Autodesk Inventor part; units mm, degrees
(part 2 of 2)
  point P149 (-121, -15)
  point P150 (-116, -14)
  point P151 (-117, -15)
  point P152 (-112, -14)
  point P153 (-113, -15)
  point P154 (-108, -14)
  point P155 (-109, -15)
  point P156 (-104, -14)
  point P157 (-105, -15)
  point P158 (-100, -14)
  point P159 (-101, -15)
  point P160 (-96, -14)
  point P161 (-97, -15)
  point P162 (-92, -14)
  point P163 (-93, -15)
  point P164 (-88, -14)
  point P165 (-89, -15)
  point P166 (-84, -14)
  point P167 (-85, -15)
  point P168 (-80, -14)
  point P169 (-81, -15)
  point P170 (-76, -14)
  point P171 (-77, -15)
  point P172 (-72, -14)
  point P173 (-73, -15)
  point P174 (-68, -14)
  point P175 (-69, -15)
  point P176 (-64, -14)
  point P177 (-65, -15)
  point P178 (-60, -14)
  point P179 (-61, -15)
  point P180 (-56, -14)
  point P181 (-57, -15)
  point P182 (-52, -14)
  point P183 (-53, -15)
  point P184 (-48, -14)
  point P185 (-49, -15)
  point P186 (-44, -14)
  point P187 (-45, -15)
  point P188 (-40, -14)
  point P189 (-41, -15)
  point P190 (-36, -14)
  point P191 (-37, -15)
  point P192 (-32, -14)
  point P193 (-33, -15)
  point P194 (-124, -17)
  point P195 (-125, -18)
  point P196 (-120, -17)
  point P197 (-121, -18)
  point P198 (-116, -17)
  point P199 (-117, -18)
  dimension "d81" = 3
  dimension "d82" = 3
  dimension "d83" = 2
  dimension "d84" = 2
  dimension "d87" = 4
  dimension "d90" = 3
  constraints: 2304 end point, 2 collinear, 2 horizontal, 2 midpoint, 2 parallel, 1 perpendicular, 1 point on circle, 1 vertical, 2868 other
  measures "d81" distance from line of L4 point (-124, -5)
  measures "d82" horizontal distance of point (-128, -22.5) point (-125, -6)
  measures "d83" distance of L1.end L2.end
  measures "d84" distance of L0.end L1.end
  measures "d87" distance of L0.start L5.start
  measures "d90" distance of L0.start L97.start
extrude "Extrusion8" cut sketch "Sketch12" against normal blind 10
sketch "Sketch13" plane through (0, 2, 0) normal (0, 1, 0) x (1, 0, 0)
  point P0 (0, 0)
sketch "Sketch15" plane through (0, 2, 0) normal (0, 1, 0) x (1, 0, 0)
  line L0 (-29, -5) -> (-27, -5)
  line L1 (-27, -5) -> (-27, -7)
  line L2 (-27, -7) -> (-29, -7)
  line L3 (-29, -7) -> (-29, -5)
  line L4 (-31, -5) -> (-31, -7) projected
  line L5 (-25, -5) -> (-23, -5)
  line L6 (-23, -5) -> (-23, -7)
  line L7 (-23, -7) -> (-25, -7)
  line L8 (-25, -7) -> (-25, -5)
  line L9 (-21, -5) -> (-19, -5)
  line L10 (-19, -5) -> (-19, -7)
  line L11 (-19, -7) -> (-21, -7)
  line L12 (-21, -7) -> (-21, -5)
  line L13 (-29, -8) -> (-27, -8)
  line L14 (-27, -8) -> (-27, -10)
  line L15 (-27, -10) -> (-29, -10)
  line L16 (-29, -10) -> (-29, -8)
  line L17 (-25, -8) -> (-23, -8)
  line L18 (-23, -8) -> (-23, -10)
  line L19 (-23, -10) -> (-25, -10)
  line L20 (-25, -10) -> (-25, -8)
  line L21 (-21, -8) -> (-19, -8)
  line L22 (-19, -8) -> (-19, -10)
  line L23 (-19, -10) -> (-21, -10)
  line L24 (-21, -10) -> (-21, -8)
  line L25 (-29, -11) -> (-27, -11)
  line L26 (-27, -11) -> (-27, -13)
  line L27 (-27, -13) -> (-29, -13)
  line L28 (-29, -13) -> (-29, -11)
  line L29 (-25, -11) -> (-23, -11)
  line L30 (-23, -11) -> (-23, -13)
  line L31 (-23, -13) -> (-25, -13)
  line L32 (-25, -13) -> (-25, -11)
  line L33 (-21, -11) -> (-19, -11)
  line L34 (-19, -11) -> (-19, -13)
  line L35 (-19, -13) -> (-21, -13)
  line L36 (-21, -13) -> (-21, -11)
  line L37 (-29, -14) -> (-27, -14)
  line L38 (-27, -14) -> (-27, -16)
  line L39 (-27, -16) -> (-29, -16)
  line L40 (-29, -16) -> (-29, -14)
  line L41 (-25, -14) -> (-23, -14)
  line L42 (-23, -14) -> (-23, -16)
  line L43 (-23, -16) -> (-25, -16)
  line L44 (-25, -16) -> (-25, -14)
  line L45 (-21, -14) -> (-19, -14)
  line L46 (-19, -14) -> (-19, -16)
  line L47 (-19, -16) -> (-21, -16)
  line L48 (-21, -16) -> (-21, -14)
  line L49 (-29, -17) -> (-27, -17)
  line L50 (-27, -17) -> (-27, -19)
  line L51 (-27, -19) -> (-29, -19)
  line L52 (-29, -19) -> (-29, -17)
  line L53 (-25, -17) -> (-23, -17)
  line L54 (-23, -17) -> (-23, -19)
  line L55 (-23, -19) -> (-25, -19)
  line L56 (-25, -19) -> (-25, -17)
  line L57 (-21, -17) -> (-19, -17)
  line L58 (-19, -17) -> (-19, -19)
  line L59 (-19, -19) -> (-21, -19)
  line L60 (-21, -19) -> (-21, -17)
  line L61 (-29, -20) -> (-27, -20)
  line L62 (-27, -20) -> (-27, -22)
  line L63 (-27, -22) -> (-29, -22)
  line L64 (-29, -22) -> (-29, -20)
  line L65 (-25, -20) -> (-23, -20)
  line L66 (-23, -20) -> (-23, -22)
  line L67 (-23, -22) -> (-25, -22)
  line L68 (-25, -22) -> (-25, -20)
  line L69 (-21, -20) -> (-19, -20)
  line L70 (-19, -20) -> (-19, -22)
  line L71 (-19, -22) -> (-21, -22)
  line L72 (-21, -22) -> (-21, -20)
  line L73 (-29, -23) -> (-27, -23)
  line L74 (-27, -23) -> (-27, -25)
  line L75 (-27, -25) -> (-29, -25)
  line L76 (-29, -25) -> (-29, -23)
  line L77 (-25, -23) -> (-23, -23)
  line L78 (-23, -23) -> (-23, -25)
  line L79 (-23, -25) -> (-25, -25)
  line L80 (-25, -25) -> (-25, -23)
  line L81 (-21, -23) -> (-19, -23)
  line L82 (-19, -23) -> (-19, -25)
  line L83 (-19, -25) -> (-21, -25)
  line L84 (-21, -25) -> (-21, -23)
  line L85 (-29, -29) -> (-27, -29)
  line L86 (-27, -27) -> (-29, -27)
  line L87 (-29, -26) -> (-27, -26)
  line L88 (-27, -26) -> (-27, -28)
  line L89 (-27, -28) -> (-29, -28)
  line L90 (-29, -28) -> (-29, -26)
  line L91 (-25, -26) -> (-23, -26)
  line L92 (-23, -26) -> (-23, -28)
  line L93 (-23, -28) -> (-25, -28)
  line L94 (-25, -28) -> (-25, -26)
  line L95 (-21, -26) -> (-19, -26)
  line L96 (-19, -26) -> (-19, -28)
  line L97 (-19, -28) -> (-21, -28)
  line L98 (-21, -28) -> (-21, -26)
  line L99 (-29, -29) -> (-27, -29)
  line L100 (-27, -29) -> (-27, -31)
  line L101 (-27, -31) -> (-29, -31)
  line L102 (-29, -31) -> (-29, -29)
  line L103 (-25, -29) -> (-23, -29)
  line L104 (-23, -29) -> (-23, -31)
  line L105 (-23, -31) -> (-25, -31)
  line L106 (-25, -31) -> (-25, -29)
  line L107 (-21, -29) -> (-19, -29)
  line L108 (-19, -29) -> (-19, -31)
  line L109 (-19, -31) -> (-21, -31)
  line L110 (-21, -31) -> (-21, -29)
  line L111 (-29, -32) -> (-27, -32)
  line L112 (-27, -32) -> (-27, -34)
  line L113 (-27, -34) -> (-29, -34)
  line L114 (-29, -34) -> (-29, -32)
  line L115 (-25, -32) -> (-23, -32)
  line L116 (-23, -32) -> (-23, -34)
  line L117 (-23, -34) -> (-25, -34)
  line L118 (-25, -34) -> (-25, -32)
  line L119 (-21, -32) -> (-19, -32)
  line L120 (-19, -32) -> (-19, -34)
  line L121 (-19, -34) -> (-21, -34)
  line L122 (-21, -34) -> (-21, -32)
  line L123 (-29, -35) -> (-27, -35)
  line L124 (-27, -35) -> (-27, -36.9954)
  line L125 (-27, -36.9954) -> (-29, -36.9954)
  line L126 (-29, -36.9954) -> (-29, -35)
  line L127 (-25, -35) -> (-23, -35)
  line L128 (-23, -35) -> (-23, -36.9954)
  line L129 (-23, -36.9954) -> (-25, -36.9954)
  line L130 (-25, -36.9954) -> (-25, -35)
  line L131 (-17, -20) -> (-15, -20)
  line L132 (-15, -20) -> (-15, -22)
  line L133 (-15, -22) -> (-17, -22)
  line L134 (-17, -22) -> (-17, -20)
  line L135 (-17, -17) -> (-15, -17)
  line L136 (-15, -17) -> (-15, -19)
  line L137 (-15, -19) -> (-17, -19)
  line L138 (-17, -19) -> (-17, -17)
  line L139 (-17, -14) -> (-15, -14)
  line L140 (-15, -14) -> (-15, -16)
  line L141 (-15, -16) -> (-17, -16)
  line L142 (-17, -16) -> (-17, -14)
  line L143 (-17, -11) -> (-15, -11)
  line L144 (-15, -11) -> (-15, -13)
  line L145 (-15, -13) -> (-17, -13)
  line L146 (-17, -13) -> (-17, -11)
  line L147 (-17, -8) -> (-15, -8)
  line L148 (-15, -8) -> (-15, -10)
  line L149 (-15, -10) -> (-17, -10)
  line L150 (-17, -10) -> (-17, -8)
  line L151 (-17, -5) -> (-15, -5)
  line L152 (-15, -5) -> (-15, -7)
  line L153 (-15, -7) -> (-17, -7)
  line L154 (-17, -7) -> (-17, -5)
  line L155 (-13, -5) -> (-11, -5)
  line L156 (-11, -5) -> (-11, -7)
  line L157 (-11, -7) -> (-13, -7)
  line L158 (-13, -7) -> (-13, -5)
  line L159 (-11, -8) -> (-13, -8)
  line L160 (-13, -8) -> (-13, -10)
  line L161 (-13, -10) -> (-11, -10)
  line L162 (-11, -10) -> (-11, -8)
  line L163 (-11, -11) -> (-13, -11)
  line L164 (-13, -11) -> (-13, -13)
  line L165 (-13, -13) -> (-11, -13)
  line L166 (-11, -13) -> (-11, -11)
  line L167 (-11, -14) -> (-13, -14)
  line L168 (-13, -14) -> (-13, -16)
  line L169 (-13, -16) -> (-11, -16)
  line L170 (-11, -16) -> (-11, -14)
  line L171 (-11, -17) -> (-13, -17)
  line L172 (-13, -17) -> (-13, -19)
  line L173 (-13, -19) -> (-11, -19)
  line L174 (-11, -19) -> (-11, -17)
  line L175 (-11, -20) -> (-13, -20)
  line L176 (-13, -20) -> (-13, -22)
  line L177 (-13, -22) -> (-11, -22)
  line L178 (-11, -22) -> (-11, -20)
  line L179 (-15, -23) -> (-17, -23)
  line L180 (-17, -23) -> (-17, -25)
  line L181 (-17, -25) -> (-15, -25)
  line L182 (-15, -25) -> (-15, -23)
  line L183 (-15, -26) -> (-17, -26)
  line L184 (-17, -26) -> (-17, -28)
  line L185 (-17, -28) -> (-15, -28)
  line L186 (-15, -28) -> (-15, -26)
  line L187 (-15, -29) -> (-17, -29)
  line L188 (-17, -29) -> (-17, -31)
  line L189 (-17, -31) -> (-15, -31)
  line L190 (-15, -31) -> (-15, -29)
  line L191 (-11, -23) -> (-13, -23)
  line L192 (-13, -23) -> (-13, -25)
  line L193 (-13, -25) -> (-11, -25)
  line L194 (-11, -25) -> (-11, -23)
  line L195 (-9, -5) -> (-7, -5)
  line L196 (-7, -5) -> (-7, -7)
  line L197 (-7, -7) -> (-9, -7)
  line L198 (-9, -7) -> (-9, -5)
  line L199 (-7, -8) -> (-9, -8)
  line L200 (-9, -8) -> (-9, -10)
  line L201 (-9, -10) -> (-7, -10)
  line L202 (-7, -10) -> (-7, -8)
  line L203 (-7, -11) -> (-9, -11)
  line L204 (-9, -11) -> (-9, -13)
  line L205 (-9, -13) -> (-7, -13)
  line L206 (-7, -13) -> (-7, -11)
  line L207 (-7, -14) -> (-9, -14)
  line L208 (-9, -14) -> (-9, -16)
  line L209 (-9, -16) -> (-7, -16)
  line L210 (-7, -16) -> (-7, -14)
  line L211 (-7, -17) -> (-9, -17)
  line L212 (-9, -17) -> (-9, -19)
  line L213 (-9, -19) -> (-7, -19)
  line L214 (-7, -19) -> (-7, -17)
  line L215 (-29, -37.9074) -> (-27, -37.9074)
  line L216 (-27, -37.9074) -> (-27, -39.9074)
  line L217 (-27, -39.9074) -> (-29, -39.9074)
  line L218 (-29, -39.9074) -> (-29, -37.9074)
  line L219 (-31, -38) -> (-31, -40) projected
  line L220 (-9, -20) -> (-7, -20)
  line L221 (-7, -20) -> (-7, -22.182)
  line L222 (-7, -22.182) -> (-9, -22.182)
  line L223 (-9, -22.182) -> (-9, -20)
  line L224 (-13, -26) -> (-11, -26)
  line L225 (-11, -26) -> (-11, -28)
  line L226 (-11, -28) -> (-13, -28)
  line L227 (-13, -28) -> (-13, -26)
  line L228 (-17, -32) -> (-15, -32)
  line L229 (-15, -32) -> (-15, -34)
  line L230 (-15, -34) -> (-17, -34)
  line L231 (-17, -34) -> (-17, -32)
  line L232 (-21, -35) -> (-19, -35)
  line L233 (-19, -35) -> (-19, -36.9954)
  line L234 (-19, -36.9954) -> (-21, -36.9954)
  line L235 (-21, -36.9954) -> (-21, -35)
  line L236 (-9, -10) -> (-9, -8)
  line L237 (-7, -8) -> (-7, -10)
  line L238 (-7, -10) -> (-9, -10)
  line L239 (-9, -8) -> (-7, -8)
  line L240 (-9, -13) -> (-9, -11)
  line L241 (-7, -11) -> (-7, -13)
  line L242 (-7, -13) -> (-9, -13)
  line L243 (-9, -11) -> (-7, -11)
  line L244 (-9, -16) -> (-9, -14)
  line L245 (-7, -14) -> (-7, -16)
  line L246 (-7, -16) -> (-9, -16)
  line L247 (-9, -14) -> (-7, -14)
  line L248 (-9, -19) -> (-9, -17)
  line L249 (-7, -17) -> (-7, -19)
  line L250 (-7, -19) -> (-9, -19)
  line L251 (-9, -17) -> (-7, -17)
  line L252 (-9, -22) -> (-9, -20)
  line L253 (-7, -20) -> (-7, -22)
  line L254 (-7, -22) -> (-9, -22)
  line L255 (-9, -20) -> (-7, -20)
  line L256 (-9, -25) -> (-9, -23)
  line L257 (-7, -23) -> (-7, -25)
  line L258 (-7, -25) -> (-9, -25)
  line L259 (-9, -23) -> (-7, -23)
  line L260 (-9, -28) -> (-9, -26)
  line L261 (-7, -26) -> (-7, -28)
  line L262 (-7, -28) -> (-9, -28)
  line L263 (-9, -26) -> (-7, -26)
  line L264 (-9, -31) -> (-9, -29)
  line L265 (-7, -29) -> (-7, -31)
  line L266 (-7, -31) -> (-9, -31)
  line L267 (-9, -29) -> (-7, -29)
  line L268 (-9, -34) -> (-9, -32)
  line L269 (-7, -32) -> (-7, -34)
  line L270 (-7, -34) -> (-9, -34)
  line L271 (-9, -32) -> (-7, -32)
  line L272 (-9, -37) -> (-9, -35)
  line L273 (-7, -35) -> (-7, -37)
  line L274 (-7, -37) -> (-9, -37)
  line L275 (-9, -35) -> (-7, -35)
  line L276 (-9, -40) -> (-9, -38)
  line L277 (-7, -38) -> (-7, -40)
  line L278 (-7, -40) -> (-9, -40)
  line L279 (-9, -38) -> (-7, -38)
  line L280 (-13, -7) -> (-13, -5)
  line L281 (-11, -5) -> (-11, -7)
  line L282 (-11, -7) -> (-13, -7)
  line L283 (-13, -5) -> (-11, -5)
  line L284 (-13, -10) -> (-13, -8)
  line L285 (-11, -8) -> (-11, -10)
  line L286 (-11, -10) -> (-13, -10)
  line L287 (-13, -8) -> (-11, -8)
  line L288 (-13, -13) -> (-13, -11)
  line L289 (-11, -11) -> (-11, -13)
  line L290 (-11, -13) -> (-13, -13)
  line L291 (-13, -11) -> (-11, -11)
  line L292 (-13, -16) -> (-13, -14)
  line L293 (-11, -14) -> (-11, -16)
  line L294 (-11, -16) -> (-13, -16)
  line L295 (-13, -14) -> (-11, -14)
  line L296 (-13, -19) -> (-13, -17)
  line L297 (-11, -17) -> (-11, -19)
  line L298 (-11, -19) -> (-13, -19)
  line L299 (-13, -17) -> (-11, -17)
  line L300 (-13, -22) -> (-13, -20)
  line L301 (-11, -20) -> (-11, -22)
  line L302 (-11, -22) -> (-13, -22)
  line L303 (-13, -20) -> (-11, -20)
  line L304 (-13, -25) -> (-13, -23)
  line L305 (-11, -23) -> (-11, -25)
  line L306 (-11, -25) -> (-13, -25)
  line L307 (-13, -23) -> (-11, -23)
  line L308 (-13, -28) -> (-13, -26)
  line L309 (-11, -26) -> (-11, -28)
  line L310 (-11, -28) -> (-13, -28)
  line L311 (-13, -26) -> (-11, -26)
  line L312 (-13, -31) -> (-13, -29)
  line L313 (-11, -29) -> (-11, -31)
  line L314 (-11, -31) -> (-13, -31)
  line L315 (-13, -29) -> (-11, -29)
  line L316 (-13, -34) -> (-13, -32)
  line L317 (-11, -32) -> (-11, -34)
  line L318 (-11, -34) -> (-13, -34)
  line L319 (-13, -32) -> (-11, -32)
  line L320 (-13, -37) -> (-13, -35)
  line L321 (-11, -35) -> (-11, -37)
  line L322 (-11, -37) -> (-13, -37)
  line L323 (-13, -35) -> (-11, -35)
  line L324 (-13, -40) -> (-13, -38)
  line L325 (-11, -38) -> (-11, -40)
  line L326 (-11, -40) -> (-13, -40)
  line L327 (-13, -38) -> (-11, -38)
  line L328 (-17, -7) -> (-17, -5)
  line L329 (-15, -5) -> (-15, -7)
  line L330 (-15, -7) -> (-17, -7)
  line L331 (-17, -5) -> (-15, -5)
  line L332 (-17, -10) -> (-17, -8)
  line L333 (-15, -8) -> (-15, -10)
  line L334 (-15, -10) -> (-17, -10)
  line L335 (-17, -8) -> (-15, -8)
  line L336 (-17, -13) -> (-17, -11)
  line L337 (-15, -11) -> (-15, -13)
  line L338 (-15, -13) -> (-17, -13)
  line L339 (-17, -11) -> (-15, -11)
  line L340 (-17, -16) -> (-17, -14)
  line L341 (-15, -14) -> (-15, -16)
  line L342 (-15, -16) -> (-17, -16)
  line L343 (-17, -14) -> (-15, -14)
  line L344 (-17, -19) -> (-17, -17)
  line L345 (-15, -17) -> (-15, -19)
  line L346 (-15, -19) -> (-17, -19)
  line L347 (-17, -17) -> (-15, -17)
  line L348 (-17, -22) -> (-17, -20)
  line L349 (-15, -20) -> (-15, -22)
  line L350 (-15, -22) -> (-17, -22)
  line L351 (-17, -20) -> (-15, -20)
  line L352 (-17, -25) -> (-17, -23)
  line L353 (-15, -23) -> (-15, -25)
  line L354 (-15, -25) -> (-17, -25)
  line L355 (-17, -23) -> (-15, -23)
  line L356 (-17, -28) -> (-17, -26)
  line L357 (-15, -26) -> (-15, -28)
  line L358 (-15, -28) -> (-17, -28)
  line L359 (-17, -26) -> (-15, -26)
  line L360 (-17, -31) -> (-17, -29)
  line L361 (-15, -29) -> (-15, -31)
  line L362 (-15, -31) -> (-17, -31)
  line L363 (-17, -29) -> (-15, -29)
  line L364 (-17, -34) -> (-17, -32)
  line L365 (-15, -32) -> (-15, -34)
  line L366 (-15, -34) -> (-17, -34)
  line L367 (-17, -32) -> (-15, -32)
  line L368 (-17, -37) -> (-17, -35)
  line L369 (-15, -35) -> (-15, -37)
  line L370 (-15, -37) -> (-17, -37)
  line L371 (-17, -35) -> (-15, -35)
  line L372 (-17, -40) -> (-17, -38)
  line L373 (-15, -38) -> (-15, -40)
  line L374 (-15, -40) -> (-17, -40)
  line L375 (-17, -38) -> (-15, -38)
  line L376 (-21, -7) -> (-21, -5)
  line L377 (-19, -5) -> (-19, -7)
  line L378 (-19, -7) -> (-21, -7)
  line L379 (-21, -5) -> (-19, -5)
  line L380 (-21, -10) -> (-21, -8)
  line L381 (-19, -8) -> (-19, -10)
  line L382 (-19, -10) -> (-21, -10)
  line L383 (-21, -8) -> (-19, -8)
  line L384 (-21, -13) -> (-21, -11)
  line L385 (-19, -11) -> (-19, -13)
  line L386 (-19, -13) -> (-21, -13)
  line L387 (-21, -11) -> (-19, -11)
  line L388 (-21, -16) -> (-21, -14)
  line L389 (-19, -14) -> (-19, -16)
  line L390 (-19, -16) -> (-21, -16)
  line L391 (-21, -14) -> (-19, -14)
  line L392 (-21, -19) -> (-21, -17)
  line L393 (-19, -17) -> (-19, -19)
  line L394 (-19, -19) -> (-21, -19)
  line L395 (-21, -17) -> (-19, -17)
  line L396 (-21, -22) -> (-21, -20)
  line L397 (-19, -20) -> (-19, -22)
  line L398 (-19, -22) -> (-21, -22)
  line L399 (-21, -20) -> (-19, -20)
  line L400 (-21, -25) -> (-21, -23)
  line L401 (-19, -23) -> (-19, -25)
  line L402 (-19, -25) -> (-21, -25)
  line L403 (-21, -23) -> (-19, -23)
  line L404 (-21, -28) -> (-21, -26)
  line L405 (-19, -26) -> (-19, -28)
  line L406 (-19, -28) -> (-21, -28)
  line L407 (-21, -26) -> (-19, -26)
  line L408 (-21, -31) -> (-21, -29)
  line L409 (-19, -29) -> (-19, -31)
  line L410 (-19, -31) -> (-21, -31)
  line L411 (-21, -29) -> (-19, -29)
  line L412 (-21, -34) -> (-21, -32)
  line L413 (-19, -32) -> (-19, -34)
  line L414 (-19, -34) -> (-21, -34)
  line L415 (-21, -32) -> (-19, -32)
  line L416 (-21, -37) -> (-21, -35)
  line L417 (-19, -35) -> (-19, -37)
  line L418 (-19, -37) -> (-21, -37)
  line L419 (-21, -35) -> (-19, -35)
  line L420 (-21, -40) -> (-21, -38)
  line L421 (-19, -38) -> (-19, -40)
  line L422 (-19, -40) -> (-21, -40)
  line L423 (-21, -38) -> (-19, -38)
  line L424 (-25, -7) -> (-25, -5)
  line L425 (-23, -5) -> (-23, -7)
  line L426 (-23, -7) -> (-25, -7)
  line L427 (-25, -5) -> (-23, -5)
  line L428 (-25, -10) -> (-25, -8)
  line L429 (-23, -8) -> (-23, -10)
  line L430 (-23, -10) -> (-25, -10)
  line L431 (-25, -8) -> (-23, -8)
  line L432 (-25, -13) -> (-25, -11)
  line L433 (-23, -11) -> (-23, -13)
  line L434 (-23, -13) -> (-25, -13)
  line L435 (-25, -11) -> (-23, -11)
  line L436 (-25, -16) -> (-25, -14)
  line L437 (-23, -14) -> (-23, -16)
  line L438 (-23, -16) -> (-25, -16)
  line L439 (-25, -14) -> (-23, -14)
  line L440 (-25, -19) -> (-25, -17)
  line L441 (-23, -17) -> (-23, -19)
  line L442 (-23, -19) -> (-25, -19)
  line L443 (-25, -17) -> (-23, -17)
  line L444 (-25, -22) -> (-25, -20)
  line L445 (-23, -20) -> (-23, -22)
  line L446 (-23, -22) -> (-25, -22)
  line L447 (-25, -20) -> (-23, -20)
  line L448 (-25, -25) -> (-25, -23)
  line L449 (-23, -23) -> (-23, -25)
  line L450 (-23, -25) -> (-25, -25)
  line L451 (-25, -23) -> (-23, -23)
  line L452 (-25, -28) -> (-25, -26)
  line L453 (-23, -26) -> (-23, -28)
  line L454 (-23, -28) -> (-25, -28)
  line L455 (-25, -26) -> (-23, -26)
  line L456 (-25, -31) -> (-25, -29)
  line L457 (-23, -29) -> (-23, -31)
  line L458 (-23, -31) -> (-25, -31)
  line L459 (-25, -29) -> (-23, -29)
  line L460 (-25, -34) -> (-25, -32)
  line L461 (-23, -32) -> (-23, -34)
  line L462 (-23, -34) -> (-25, -34)
  line L463 (-25, -32) -> (-23, -32)
  line L464 (-25, -37) -> (-25, -35)
  line L465 (-23, -35) -> (-23, -37)
  line L466 (-23, -37) -> (-25, -37)
  line L467 (-25, -35) -> (-23, -35)
  line L468 (-25, -40) -> (-25, -38)
  line L469 (-23, -38) -> (-23, -40)
  line L470 (-23, -40) -> (-25, -40)
  line L471 (-25, -38) -> (-23, -38)
  line L472 (-29, -7) -> (-29, -5)
  line L473 (-27, -5) -> (-27, -7)
  line L474 (-27, -7) -> (-29, -7)
  line L475 (-29, -5) -> (-27, -5)
  line L476 (-29, -10) -> (-29, -8)
  line L477 (-27, -8) -> (-27, -10)
  line L478 (-27, -10) -> (-29, -10)
  line L479 (-29, -8) -> (-27, -8)
  line L480 (-29, -13) -> (-29, -11)
  line L481 (-27, -11) -> (-27, -13)
  line L482 (-27, -13) -> (-29, -13)
  line L483 (-29, -11) -> (-27, -11)
  line L484 (-29, -16) -> (-29, -14)
  line L485 (-27, -14) -> (-27, -16)
  line L486 (-27, -16) -> (-29, -16)
  line L487 (-29, -14) -> (-27, -14)
  line L488 (-29, -19) -> (-29, -17)
  line L489 (-27, -17) -> (-27, -19)
  line L490 (-27, -19) -> (-29, -19)
  line L491 (-29, -17) -> (-27, -17)
  line L492 (-29, -22) -> (-29, -20)
  line L493 (-27, -20) -> (-27, -22)
  line L494 (-27, -22) -> (-29, -22)
  line L495 (-29, -20) -> (-27, -20)
  line L496 (-29, -25) -> (-29, -23)
  line L497 (-27, -23) -> (-27, -25)
  line L498 (-27, -25) -> (-29, -25)
  line L499 (-29, -23) -> (-27, -23)
  line L500 (-29, -28) -> (-29, -26)
  line L501 (-27, -26) -> (-27, -28)
  line L502 (-27, -28) -> (-29, -28)
  line L503 (-29, -26) -> (-27, -26)
  line L504 (-29, -31) -> (-29, -29)
  line L505 (-27, -29) -> (-27, -31)
  line L506 (-27, -31) -> (-29, -31)
  line L507 (-29, -29) -> (-27, -29)
  line L508 (-29, -34) -> (-29, -32)
  line L509 (-27, -32) -> (-27, -34)
  line L510 (-27, -34) -> (-29, -34)
  line L511 (-29, -32) -> (-27, -32)
  line L512 (-29, -37) -> (-29, -35)
  line L513 (-27, -35) -> (-27, -37)
  line L514 (-27, -37) -> (-29, -37)
  line L515 (-29, -35) -> (-27, -35)
  line L516 (-29, -40) -> (-29, -38)
  line L517 (-27, -38) -> (-27, -40)
  line L518 (-27, -40) -> (-29, -40)
  line L519 (-29, -38) -> (-27, -38)
  point P0 (-31, -6)
  point P1 (-29, -6)
  point P2 (-25, -6)
  point P3 (-21, -6)
  point P4 (-29, -9)
  point P5 (-25, -9)
  point P6 (-21, -9)
  point P7 (-29, -12)
  point P8 (-25, -12)
  point P9 (-21, -12)
  point P10 (-29, -15)
  point P11 (-25, -15)
  point P12 (-21, -15)
  point P13 (-29, -18)
  point P14 (-25, -18)
  point P15 (-21, -18)
  point P16 (-29, -21)
  point P17 (-25, -21)
  point P18 (-21, -21)
  point P19 (-29, -24)
  point P20 (-25, -24)
  point P21 (-21, -24)
  point P22 (-29, -24)
  point P23 (-28, -25)
  point P24 (-28, -27)
  point P25 (-29, -27)
  point P26 (-25, -27)
  point P27 (-21, -27)
  point P28 (-29, -30)
  point P29 (-25, -30)
  point P30 (-21, -30)
  point P31 (-29, -33)
  point P32 (-25, -33)
  point P33 (-21, -33)
  point P34 (-28, -35)
  point P35 (-28, -34)
  point P36 (-17, -6)
  point P37 (-17, -21)
  point P38 (-15, -21)
  point P39 (-7, -11)
  point P40 (-7, -14)
  point P41 (-7, -17)
  point P42 (-7, -20)
  point P43 (-7, -23)
  point P44 (-7, -26)
  point P45 (-7, -29)
  point P46 (-7, -32)
  point P47 (-7, -35)
  point P48 (-7, -38)
  point P49 (-7, -41)
  point P50 (-11, -11)
  point P51 (-11, -14)
  point P52 (-11, -17)
  point P53 (-11, -20)
  point P54 (-11, -23)
  point P55 (-11, -26)
  point P56 (-11, -29)
  point P57 (-11, -32)
  point P58 (-11, -35)
  point P59 (-11, -38)
  point P60 (-11, -41)
  point P61 (-15, -8)
  point P62 (-15, -11)
  point P63 (-15, -14)
  point P64 (-15, -17)
  point P65 (-15, -20)
  point P66 (-15, -23)
  point P67 (-15, -26)
  point P68 (-15, -29)
  point P69 (-15, -32)
  point P70 (-15, -35)
  point P71 (-15, -38)
  point P72 (-15, -41)
  point P73 (-19, -8)
  point P74 (-19, -11)
  point P75 (-19, -14)
  point P76 (-19, -17)
  point P77 (-19, -20)
  point P78 (-19, -23)
  point P79 (-19, -26)
  point P80 (-19, -29)
  point P81 (-19, -32)
  point P82 (-19, -35)
  point P83 (-19, -38)
  point P84 (-19, -41)
  point P85 (-23, -8)
  point P86 (-23, -11)
  point P87 (-23, -14)
  point P88 (-23, -17)
  point P89 (-23, -20)
  point P90 (-23, -23)
  point P91 (-23, -26)
  point P92 (-23, -29)
  point P93 (-23, -32)
  point P94 (-23, -35)
  point P95 (-23, -38)
  point P96 (-23, -41)
  point P97 (-27, -8)
  point P98 (-27, -11)
  point P99 (-27, -14)
  point P100 (-27, -17)
  point P101 (-27, -20)
  point P102 (-27, -23)
  point P103 (-27, -26)
  point P104 (-27, -29)
  point P105 (-27, -32)
  point P106 (-27, -35)
  point P107 (-27, -38)
  point P108 (-27, -41)
  dimension "d98" = 2
  dimension "d99" = 2
  dimension "d100" = 2
  dimension "d101" = 0
  dimension "d104" = 4
  dimension "d107" = 3
  dimension "d110" = 2
  dimension "d112" = 4
  dimension "d113" = 0
  dimension "d115" = 2
  dimension "d116" = 1
  dimension "d118" = 2
  dimension "d119" = 2
  dimension "d122" = 2
  dimension "d123" = 2
  dimension "d124" = 2
  dimension "d125" = 2
  dimension "d126" = 2
  dimension "d127" = 2
  dimension "d128" = 2
  dimension "d129" = 2
  dimension "d130" = 1
  dimension "d155" = 3
  dimension "d158" = 4
  constraints: 1036 end point, 59 parallel, 36 point on line, 32 horizontal, 29 perpendicular, 10 midpoint, 4 collinear, 2 vertical, 896 other
  measures "d98" distance of L0.end L1.end
  measures "d99" distance of L1.end L2.end
  measures "d100" distance between parallel lines of L3 L4
  measures "d101" vertical distance of point (-31, -6) point (-29, -6)
  measures "d104" distance of L0.start L5.start
  measures "d107" distance of L0.start L13.start
  measures "d110" distance of L85.end L86.start
  measures "d112" distance of point (-29, -24) point (-29, -28)
  measures "d113" horizontal distance of point (-28, -25) point (-28, -27)
  measures "d115" distance of L127.start L127.end
  measures "d116" distance of point (-28, -35) point (-28, -34)
  measures "d118" distance between parallel lines of L158 L152
  measures "d119" distance from line of point (-17, -6) L10
  measures "d122" distance of L156.end L157.end
  measures "d123" distance of L155.end L156.end
  measures "d124" distance between parallel lines of L156 L198
  measures "d125" distance of L195.start L195.end
  measures "d126" distance of L215.start L215.end
  measures "d127" distance of L217.end L215.start
  measures "d128" distance between parallel lines of L219 L218
  measures "d129" distance of L226.end L224.start
  measures "d130" distance between parallel lines of L193 L224
  measures "d155" distance of L197.end L236.start
  measures "d158" distance of L197.end L280.start
extrude "Extrusion9" cut sketch "Sketch15" against normal blind 10 contours L0 L1 L2 L3 | L5 L6 L7 L8 | L9 L10 L11 L12 | L13 L14 L15 L16 | L17 L18 L19 L20 | L21 L22 L23 L24 | L25 L26 L27 L28 | L29 L30 L31 L32 | L33 L34 L35 L36 | L37 L38 L39 L40 | L41 L42 L43 L44 | L45 L46 L47 L48 | L49 L50 L51 L52 | L53 L54 L55 L56 | L57 L58 L59 L60 | L61 L62 L63 L64 | L65 L66 L67 L68 | L69 L70 L71 L72 | L73 L74 L75 L76 | L77 L78 L79 L80 | L81 L82 L83 L84 | L85 L100 L101 L102 | L88 L89 L90 L86 | L86 L90 L87 L88 | L91 L92 L93 L94 | L95 L96 L97 L98 | L103 L104 L105 L106 | L107 L108 L109 L110 | L111 L112 L113 L114 | L115 L116 L117 L118 | L119 L120 L121 L122 | L123 L124 L125 L126 | L127 L128 L129 L130 | L131 L132 L133 L134 | L135 L136 L137 L138 | L139 L140 L141 L142 | L143 L144 L145 L146 | L147 L148 L149 L150 | L151 L152 L153 L154 | L155 L156 L157 L158 | L162 L161 L160 L159 | L166 L165 L164 L163 | L170 L169 L168 L167 | L174 L173 L172 L171 | L178 L177 L176 L175 | L182 L181 L180 L179 | L186 L185 L184 L183 | L190 L189 L188 L187 | L194 L193 L192 L191 | L195 L196 L197 L198 | L202 L201 L200 L199 | L206 L205 L204 L203 | L210 L209 L208 L207 | L214 L213 L212 L211 | L215 L216 L519 L218 | L519 L216 L217 L218 | L220 L221 L254 L223 | L254 L221 L222 L223 | L224 L225 L226 L227 | L228 L229 L230 L231 | L232 L233 L234 L235 | L256 L259 L257 L258 | L312 L315 L313 L314 | L468 L471 L469 L470
sketch "Sketch20" plane through (0, 2, 0) normal (0, 1, 0) x (1, 0, 0)
  line L0 (-125, -2) -> (-2, -2) projected
  arc A0 (-7, -22.182) -> (-2, -4.6897) centre (-44.7799, -1.9222) ccw projected
  line L1 (-2, -2) -> (-5, -2)
  line L2 (-5, -2) -> (-5, -17.9015)
  line L3 (-2, -4.6897) -> (-2, -2)
  line L4 (-7, -5) -> (-7, -7) projected
  arc A1 (-5, -17.9015) -> (-2, -4.6897) centre (-44.7799, -1.9222) ccw
  point P0 (0, 0)
  dimension "d138" = 2
  constraints: 6 end point, 4 point on circle, 1 centre point, 1 concentric, 1 horizontal, 1 parallel, 1 perpendicular
  measures "d138" distance between parallel lines of L2 L4
extrude "Extrusion12" add sketch "Sketch20" along normal blind 13
sketch "Sketch21" plane through (0, 15, 0) normal (0, 1, 0) x (1, 0, 0)
  circle A0 centre (-2, -3) radius 1
  line L0 (-5, -2) -> (-5, -17.9015) projected
  line L1 (0, 0) -> (-125, 0) projected
  circle A1 centre (-132, -13) radius 1
  line L2 (-135, -10) -> (-135, -35) projected
  circle A2 centre (-132, -32) radius 1
  line L3 (-125, -45) -> (-32.5163, -45) projected
  line L4 (0, -2.8444) -> (0, 0) projected
  dimension "d141" = 2
  dimension "d142" = 3
  dimension "d143" = 3
  dimension "d144" = 2
  dimension "d145" = 3
  dimension "d146" = 13
  dimension "d147" = 2
  dimension "d148" = 3
  dimension "d149" = 13
  dimension "d152" = 2
  constraints: 3 centre point
  measures "d141" diameter of A0
  measures "d142" distance from line of L0 A0.centre
  measures "d143" distance from line of L1 A0.centre
  measures "d144" diameter of A1
  measures "d145" distance from line of L2 A1.centre
  measures "d146" vertical distance of L1.end A1.centre
  measures "d147" diameter of A2
  measures "d148" distance from line of L2 A2.centre
  measures "d149" distance from line of A2.centre L3
  measures "d152" distance from line of L4 A0.centre
extrude "Extrusion13" cut sketch "Sketch21" against normal blind 3
body "Solid2"
